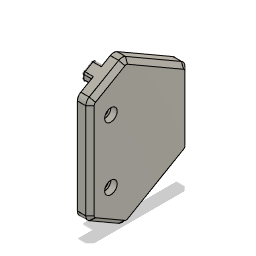
Full Clamp (Autodesk Fusion 360 design; units mm, degrees)
Autodesk Fusion 360 part; units mm, degrees
sketch "Sketch1" plane through (0, 0, 0) normal (1, 0, 0) x (0, 0, -1)
  line L0 (17.3205, -30) -> (34.641, 0)
  line L1 (34.641, 0) -> (17.3205, 30)
  line L2 (17.3205, 30) -> (-17.3205, 30)
  line L3 (-17.3205, 30) -> (-34.641, 0)
  line L4 (-34.641, 0) -> (-17.3205, -30)
  line L5 (-17.3205, -30) -> (17.3205, -30)
  line L6 (-17.3205, 30) -> (2.6795, 30) construction
  line L7 (2.6795, 30) -> (2.6795, -30) construction
  line L8 (2.6795, -30) -> (-17.3205, -30) construction
  line L9 (-17.3205, -30) -> (-17.3205, 30) construction
  line L10 (-17.3205, 0) -> (2.6795, 0)
  line L11 (-17.3205, 30) -> (-17.3205, 0)
  line L12 (-17.3205, 0) -> (-17.3205, -30)
  line L13 (-17.3205, 0) -> (2.6795, -30) construction
  line L14 (-17.3205, 0) -> (2.6795, 30) construction
  circle A0 centre (-7.3205, 15) radius 1.7
  circle A1 centre (-7.3205, -15) radius 1.7
  circle A2 centre (-7.3205, 15) radius 3
  circle A3 centre (-7.3205, -15) radius 3
  line L15 (-7.3205, 30) -> (-7.3205, -30) construction
  line L16 (-4.4205, 25) -> (-10.2205, 25)
  line L17 (-10.2205, 25) -> (-10.2205, 35)
  line L18 (-10.2205, 35) -> (-4.4205, 35)
  line L19 (-4.4205, 35) -> (-4.4205, 25)
  line L20 (-4.4205, 25) -> (-10.2205, 35) construction
  line L21 (-10.2205, 25) -> (-4.4205, 35) construction
  line L22 (-4.4205, -35) -> (-10.2205, -35)
  line L23 (-10.2205, -35) -> (-10.2205, -25)
  line L24 (-10.2205, -25) -> (-4.4205, -25)
  line L25 (-4.4205, -25) -> (-4.4205, -35)
  line L26 (-4.4205, -35) -> (-10.2205, -25) construction
  line L27 (-10.2205, -35) -> (-4.4205, -25) construction
  line L28 (-17.3205, 30) -> (-17.3205, -30)
  line L29 (-17.3205, -30) -> (-21.5905, -30)
  line L30 (-21.5905, -30) -> (-21.5905, 30)
  line L31 (-21.5905, 30) -> (-17.3205, 30)
  line L32 (30, -17.3205) -> (30, 17.3205)
  line L33 (30, 17.3205) -> (0, 34.641)
  line L34 (0, 34.641) -> (-30, 17.3205)
  line L35 (-30, 17.3205) -> (-30, -17.3205)
  line L36 (-30, -17.3205) -> (0, -34.641)
  line L37 (0, -34.641) -> (30, -17.3205)
  point P0 (-7.3205, 30)
  point P1 (-7.3205, -30)
  dimension "d1" = 30
  dimension "d2" = 20
  dimension "d3" = 3.4
  dimension "d4" = 3.4
  dimension "d5" = 6
  dimension "d6" = 6
  dimension "d7" = 5.8
  dimension "d8" = 10
  dimension "d9" = 5.8
  dimension "d10" = 10
  dimension "d11" = 4.27
  dimension "d12" = 30
  constraint perpendicular L6 L7
  constraint parallel L6 L8
  constraint parallel L7 L9
  constraint coincident L2 L6.end
  constraint midpoint L9 L10.start
  constraint midpoint L7 L10.end
  constraint midpoint L14 A0.centre
  constraint midpoint L13 A1.centre
  constraint concentric A0 A2
  constraint concentric A1 A3
  constraint midpoint L6 P0
  constraint midpoint L8 P1
  constraint horizontal L16
  constraint perpendicular L16 L17
  constraint parallel L16 L18
  constraint parallel L17 L19
  constraint coincident L20 P0
  constraint coincident L21 P0
  constraint coincident P0 L15.start
  constraint horizontal L22
  constraint perpendicular L22 L23
  constraint parallel L22 L24
  constraint parallel L23 L25
  constraint coincident L26 P1
  constraint coincident L27 P1
  constraint coincident P1 L15.end
  constraint perpendicular L28 L29
  constraint parallel L28 L30
  constraint parallel L29 L31
  constraint parallel L30 L35
  measures "d1" distance of origin L5
  measures "d2" distance of L2.end L6.end
  measures "d3" diameter of A0
  measures "d4" diameter of A1
  measures "d5" diameter of A2
  measures "d6" diameter of A3
  measures "d7" distance of L17.end L18.end
  measures "d8" distance of L16.end L17.end
  measures "d9" distance of L23.end L24.end
  measures "d10" distance of L22.end L23.end
  measures "d11" distance of L2.end L30.end
  measures "d12" distance of origin L37
extrude "Extrude1" add sketch "Sketch1" along normal blind 6 contours L0 L1 L2 L5 L11 L12 L16 L17 L19 L23 L24 L25 L28 L32 L33 L34 L36 L37 | L0 L32 L37 | L5 L25 L36 L37 | L5 L25 L36 | L5 L23 L24 L25 L36 | L1 L32 L33 | L2 L19 L33 L34 | L2 L16 L17 L19 L34 | L2 L19 L34
extrude "Extrude2" add sketch "Sketch1" against normal blind 5 contours L5 L25 L36 | L5 L23 L24 L25 L36 | L2 L16 L17 L19 L34 | L2 L19 L34
extrude "Extrude3" add sketch "Sketch1" along normal blind 3 contours A2 | A3
fillet "Fillet1" radius 3.25 6 edges at (3, -34.641, 0) (3, -17.3205, -30) (3, 17.3205, -30) (3, 34.641, 0) (3, 24.641, 17.3205) (3, -24.641, 17.3205)
chamfer "Chamfer1" distance 2 angle 45 12 edges at (6, -25.9808, -15) (6, -17.0691, -29.5646) (6, 0, -30) (6, 17.0691, -29.5646) (6, 25.9808, -15) (6, 34.1382, 0) (6, 29.641, 8.6603) (6, 24.3896, 16.8851) (6, 0, 17.3205) (6, -24.3896, 16.8851) (6, -29.641, 8.6603) (6, -34.1382, 0)
fillet "Fillet2" radius 1 9 edges at (-2.5, 25, 4.4205) (-2.5, 25, 10.2205) (-2.5, -32.0888, 4.4205) (-2.5, -28.7402, 10.2205) (-2.5, -25, 10.2205) (-2.5, -25, 4.4205) (-5, -25, 7.3205) (-2.5, 28.7402, 10.2205) (-2.5, 32.0888, 4.4205) 2 faces at (-5, -28.6097, 6.3538) (-5, 28.6097, 6.3538)
